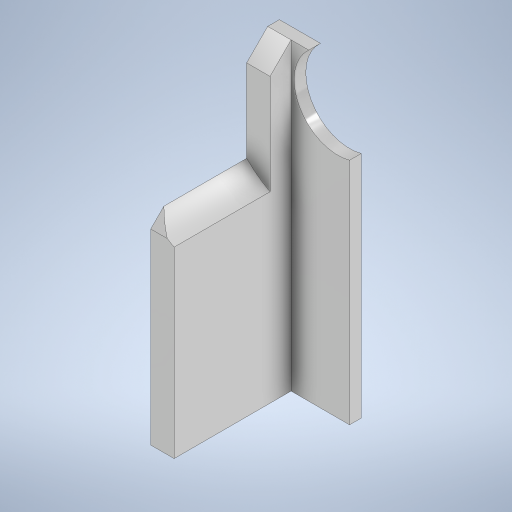
# Autodesk Inventor part: SecondSpindleOsnova
Saved by Autodesk Inventor 2024 (Build 280153000, 153)
## iProperties
Created: 2023-11-12
Part Number: SecondSpindleOsnova
Material: Aluminum 6061-AHC
Document SubType Name: Modeling
Designer: KirikDK
Mass: 2004.75 g
Surface Area: 784 cm^2
Volume: 742.5 cm^3
Density: 2.7 g/cm^3
Appearance: Aluminum - Dark
Author: KirikDK
Autodesk Inventor part; units mm, degrees
ref_plane "YZ Plane" through (0, 0, 0) normal (1, 0, 0) x (0, 1, 0)
ref_plane "XZ Plane" through (0, 0, 0) normal (0, 1, 0) x (-1, 0, 0)
ref_plane "XY Plane" through (0, 0, 0) normal (0, 0, 1) x (1, 0, 0)
sketch "Sketch1" plane through (0, 0, 0) normal (0, 1, 0) x (-1, 0, 0)
  line L0 (-3.913, 66.9565) -> (-23.913, 66.9565)
  line L1 (-23.913, 66.9565) -> (-23.913, -43.0435)
  line L2 (-23.913, -43.0435) -> (-3.913, -43.0435)
  line L3 (-3.913, -43.0435) -> (-3.913, 66.9565)
  line L4 (53.6957, 6.9565) -> (-3.913, 6.9565)
  line L5 (-3.913, 6.9565) -> (-3.913, -18.0435)
  line L6 (-3.913, -18.0435) -> (48.6957, -18.0435)
  point P0 (0, 0)
  dimension "d0" = 110
  dimension "d1" = 20
  dimension "d3" = 60
  constraints: 14 end point, 3 parallel, 2 horizontal, 2 perpendicular, 1 point on line
  measures "d0" distance of L0.end L1.end
  measures "d1" distance of L1.end L2.end
  measures "d3" distance between parallel lines of L0 L4
extrude "Extrusion1" add sketch "Sketch1" along normal blind 260
chamfer "Chamfer1" distance 100 angle 45 1 edges at (13.913, 260, 66.9565)
sketch "Sketch2" plane through (23.913, 0, 66.9565) normal (1, 0, 0) x (0, 0, -1)
  line L0 (110, 0) -> (110, 260) projected
  line L1 (110, 0) -> (0, 0) projected
  line L2 (110, 260) -> (100, 260)
  line L3 (100, 260) -> (100, 0)
  line L4 (100, 0) -> (110, 0)
  line L5 (110, 0) -> (110, 260)
  point P0 (100, 260)
  dimension "d9" = 10
  constraints: 8 end point, 2 parallel, 1 horizontal, 1 perpendicular, 1 point on line
  measures "d9" distance of L0.end L2.end
extrude "Extrusion2" add sketch "Sketch2" along normal blind 50
sketch "Sketch4" plane through (3.913, 0, 66.9565) normal (0, 0, 1) x (1, 0, 0)
  circle A0 centre (60, 232) radius 85.3728
  point P0 (-3.913, 0)
  constraints: 1 centre point
extrude "Extrusion4" cut sketch "Sketch4" against normal blind 82
sketch "Sketch5" plane through (3.913, 0, -15.0435) normal (0, 0, 1) x (1, 0, 0)
  arc A0 (0, 171.2669) -> (14.125, 160) centre (60, 232) ccw projected
  circle A1 centre (60, 232) radius 37.4531
  point P0 (-3.913, 0)
  point P1 (20, 162.1931)
  constraints: 1 centre point, 1 coincident
extrude "Extrusion5" cut sketch "Sketch5" against normal blind 82
body "Solid1"
